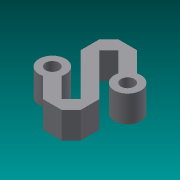
# Autodesk Inventor part: Sawaiz Logo Ribbon 3
Saved by Autodesk Inventor 2015 (Build 190159000, 159)
## iProperties
Created: 2015-06-22
Part Number: Sawaiz Logo Ribbon 3
Material: Generic
Document SubType Name: Modeling
Designer: Sawaiz Syed
Density: 1 g/cm^3
Appearance: Default
Author: Sawaiz Syed
Autodesk Inventor part; units mm, degrees
ref_plane "YZ Plane" through (0, 0, 0) normal (1, 0, 0) x (0, 1, 0)
ref_plane "XZ Plane" through (0, 0, 0) normal (0, 1, 0) x (-1, 0, 0)
ref_plane "XY Plane" through (0, 0, 0) normal (0, 0, 1) x (1, 0, 0)
sketch "Sketch1" plane through (0, 0, 0) normal (0, 0, 1) x (1, 0, 0)
  circle A0 centre (0, 0) radius 2.5
  circle A1 centre (0, 0) radius 5
  line L0 (-1.7678, -1.7678) -> (-12.3744, 8.8388)
  line L1 (-12.3744, 8.8388) -> (-15.9099, 5.3033)
  line L2 (-15.9099, 5.3033) -> (0, -10.6066)
  line L3 (0, -10.6066) -> (0, -17.6777)
  line L4 (0, -17.6777) -> (-3.5355, -21.2132)
  line L5 (-10.6066, -21.2132) -> (-21.2132, -10.6066)
  line L6 (1.7678, 1.7678) -> (-8.8388, 12.3744)
  line L7 (-15.9099, 12.3744) -> (-19.4454, 8.8388)
  line L8 (-19.4454, 8.8388) -> (-19.4454, 1.7678)
  line L9 (-19.4454, 1.7678) -> (-3.5355, -14.1421)
  line L10 (-3.5355, -14.1421) -> (-7.0711, -17.6777)
  line L11 (-7.0711, -17.6777) -> (-17.6777, -7.0711)
  line L12 (-17.6777, -7.0711) -> (-21.2132, -10.6066)
  line L13 (-1.7678, -1.7678) -> (1.7678, 1.7678)
  circle A2 centre (-19.4454, -8.8388) radius 2.5
  circle A3 centre (-19.4454, -8.8388) radius 5
  line L14 (-15.9099, 12.3744) -> (-8.8388, 12.3744)
  line L15 (-10.6066, -21.2132) -> (-3.5355, -21.2132)
  dimension "d0" = 5
  dimension "d1" = 10
  dimension "d3" = 90
  dimension "d6" = 135
  dimension "d7" = 135
  dimension "d8" = 90
  dimension "d9" = 5
  dimension "d12" = 10
  dimension "d13" = 15
  dimension "d14" = 15
  dimension "d31" = 7.0711
  dimension "d32" = 15
  dimension "d33" = 7.0711
  dimension "d34" = 15
  dimension "d35" = 7.0711
  dimension "d36" = 7.0711
  dimension "d37" = 5
  dimension "d38" = 90
  dimension "d39" = 135
  dimension "d40" = 5
  dimension "d41" = 5
  constraints: 32 end point, 4 centre point, 4 parallel, 3 coincident, 3 tangent, 2 horizontal, 2 perpendicular, 2 point on circle, 1 midpoint, 1 vertical
  measures "d0" diameter of A0
  measures "d1" diameter of A1
  measures "d3" angle of L1 L0
  measures "d6" angle of L2 L3
  measures "d7" angle of L3 L4
  measures "d8" angle of L4 L5
  measures "d9" distance of L11.end L5.end
  measures "d12" diameter of A3
  measures "d13" distance of L0.start L0.end
  measures "d14" distance of L10.end L11.end
  measures "d31" distance of L7.start L6.end
  measures "d32" distance of L6.start L6.end
  measures "d33" distance of L5.start L4.end
  measures "d34" distance of L5.start L5.end
  measures "d35" distance of L7.end L8.end
  measures "d36" distance of L2.end L3.end
  measures "d37" distance between parallel lines of L9 L2
  measures "d38" angle of L2 L1
  measures "d39" angle of L8 L7
  measures "d40" distance of L0.end L1.end
  measures "d41" distance of L9.end L10.end
extrude "Extrusion8" add sketch "Sketch1" along normal blind 10 contours A0 L6 A1 L0 | A0 L0 A1 L6 | A1 L0 L1 L2 L3 L4 L15 L5 A3 L11 L10 L9 L8 L7 L14 L6 | A3 L5 A2 L11 | L11 A2 L5 A3 | A2 L12 picked at (-19.5108, -9.6696)
sketch "Sketch5" plane through (0, 0, 10) normal (0, 0, 1) x (1, 0, 0)
  line L0 (-1.2941, 4.8296) -> (-8.8388, 12.3744) projected
  line L1 (-8.8388, 12.3744) -> (-15.9099, 12.3744) projected
  line L2 (-15.9099, 12.3744) -> (-19.4454, 8.8388) projected
  line L3 (-19.4454, 8.8388) -> (-19.4454, 1.7678) projected
  line L4 (-19.4454, 1.7678) -> (-3.5355, -14.1421) projected
  line L5 (-3.5355, -14.1421) -> (-7.0711, -17.6777) projected
  line L6 (-7.0711, -17.6777) -> (-14.6158, -10.1329) projected
  arc A0 (-14.6158, -10.1329) -> (-18.1513, -13.6685) centre (-19.4454, -8.8388) ccw projected
  line L7 (-18.1513, -13.6685) -> (-10.6066, -21.2132) projected
  line L8 (-10.6066, -21.2132) -> (-3.5355, -21.2132) projected
  line L9 (-3.5355, -21.2132) -> (0, -17.6777) projected
  line L10 (0, -17.6777) -> (0, -10.6066) projected
  line L11 (0, -10.6066) -> (-15.9099, 5.3033) projected
  line L12 (-15.9099, 5.3033) -> (-12.3744, 8.8388) projected
  line L13 (-12.3744, 8.8388) -> (-4.8296, 1.2941) projected
  arc A1 (-4.8296, 1.2941) -> (-1.2941, 4.8296) centre (0, 0) ccw projected
  line L14 (-21.2132, -10.6066) -> (-17.6777, -7.0711) projected
  arc A2 (-17.6777, -7.0711) -> (-21.2132, -10.6066) centre (-19.4454, -8.8388) ccw projected
  circle A3 centre (0, 0) radius 2.5 projected
  circle A4 centre (-19.4454, -8.8388) radius 2.5
  constraints: 1 centre point, 1 coincident, 1 concentric
extrude "Extrusion9" cut sketch "Sketch5" against normal blind 10 contours L14 A4
equation "\"d1\" = 2 * d0"
equation "\"d9\" = d0"
equation "\"d12\" = d1"
equation "\"d13\" = 3 * d0"
equation "\"d14\" = d13"
body "Solid5"
